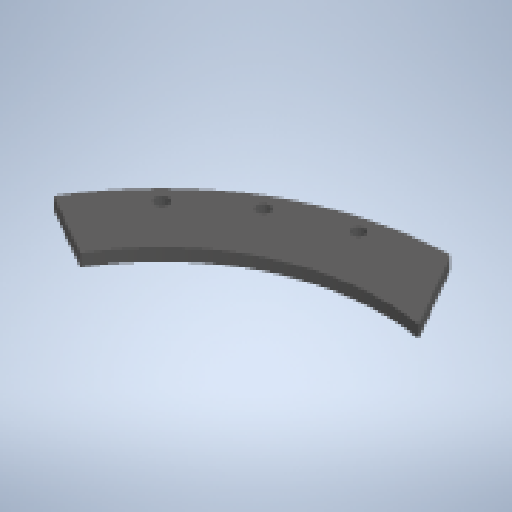
# Autodesk Inventor part: waist_side_cover
Saved by Autodesk Inventor 2024.1 (Build 281209000, 209)
## iProperties
Created: 2024-02-14
Part Number: waist_side_cover
Material: 一般
Document SubType Name: Modeling
Designer: hibik
Density: 1 g/cm^3
Appearance: 既定
Author: hibik
Autodesk Inventor part; units mm, degrees
ref_plane "YZ Plane" through (0, 0, 0) normal (1, 0, 0) x (0, 1, 0)
ref_plane "XZ Plane" through (0, 0, 0) normal (0, 1, 0) x (-1, 0, 0)
ref_plane "XY Plane" through (0, 0, 0) normal (0, 0, 1) x (1, 0, 0)
sketch "スケッチ1" plane through (0, 0, 0) normal (0, 1, 0) x (-1, 0, 0)
  circle A0 centre (0, 0) radius 27.5
  line L0 (13, 12.85) -> (-13, 12.85)
  line L1 (-13, 12.85) -> (-13, -12.85)
  line L2 (-13, -12.85) -> (13, -12.85)
  line L3 (13, -12.85) -> (13, 12.85)
  circle A1 centre (0, 0) radius 32.5 construction
  circle A2 centre (0, 0) radius 36.5
  line L4 (0, 0) -> (18.4986, -32.0406)
  line L5 (0, 0) -> (31.6099, -18.25)
  line L6 (-13, -12.85) -> (0.651, -36.4942)
  line L7 (13.2, 12.8507) -> (13.2, -12.85)
  line L8 (13.2, -12.85) -> (13, -12.85)
  circle A3 centre (0, 0) radius 34.5 construction
  circle A4 centre (24.3952, -24.3952) radius 0.8
  circle A5 centre (8.9293, -33.3244) radius 0.8
  circle A6 centre (17.25, -29.8779) radius 0.8
  line L9 (0, 0) -> (24.3952, -24.3952) construction
  line L10 (0, 0) -> (8.9293, -33.3244) construction
  point P0 (13, 0)
  point P1 (0, 12.85)
  point P2 (13, -34.1065)
  point P3 (-13, -34.1065)
  point P4 (28.1458, -16.25)
  point P5 (13, -7.5056)
  point P6 (18.25, -31.6099)
  point P7 (16.25, -28.1458)
  point P8 (23.8157, -13.75)
  point P9 (-4.7839, -27.0807)
  point P10 (-1.6802, -32.4565)
  point P11 (13.2, -7.621)
  dimension "d0" = 55
  dimension "d1" = 12.85
  dimension "d2" = 26
  dimension "d3" = 5
  dimension "d4" = 4
  dimension "d11" = 60
  dimension "d12" = 30
  dimension "d16" = 0.2
  dimension "d19" = 2
  dimension "d20" = 1.6
  dimension "d21" = 1.6
  dimension "d22" = 1.6
  dimension "d23" = 15
  dimension "d24" = 15
  constraints: 22 end point, 7 centre point, 7 point on circle, 5 coincident, 3 parallel, 2 midpoint, 2 perpendicular, 1 concentric, 1 horizontal, 1 horizontal alignment, 1 point on line, 1 vertical alignment
  measures "d0" diameter of A0
  measures "d1" distance from line of L2 point (0, 0)
  measures "d2" distance of L0.start L0.end
  measures "d3" radial gap between concentric circles of A1 A0
  measures "d4" radial gap between concentric circles of A2 A1
  measures "d11" angle of L2 L4
  measures "d12" angle of L5 L4
  measures "d16" distance between parallel lines of L7 L3
  measures "d19" radial gap between concentric circles of A2 A3
  measures "d20" diameter of A4
  measures "d21" diameter of A5
  measures "d22" diameter of A6
  measures "d23" angle of L4 L9
  measures "d24" angle of L10 L4
extrude "押し出し4" add sketch "スケッチ1" along normal blind 1.5 contours A0 L4 A6 A2 L6 | L5 A2 L4 A6 A0
equation "\"d23\" = 0.5 * d12"
equation "\"d24\" = d23"
